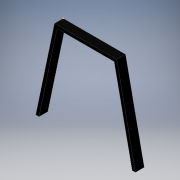
# Autodesk Inventor part: leg
Saved by Autodesk Inventor 2019 (Build 230136000, 136)
## iProperties
Created: 2019-08-11
Part Number: leg
Material: Steel, Galvanized
Document SubType Name: Modeling
Designer: Alex
Density: 7.85 g/cm^3
Appearance: Galvanized
Author: Alex
Autodesk Inventor part; units mm, degrees
ref_plane "YZ Plane" through (0, 0, 0) normal (1, 0, 0) x (0, 1, 0)
ref_plane "XZ Plane" through (0, 0, 0) normal (0, 1, 0) x (-1, 0, 0)
ref_plane "XY Plane" through (0, 0, 0) normal (0, 0, 1) x (1, 0, 0)
sketch "Sketch1" plane through (0, 0, 0) normal (1, 0, 0) x (0, 1, 0)
  point P0 (0, 0)
sketch "Sketch2" plane through (0, 0, 0) normal (0, 0, 1) x (1, 0, 0)
  line L0 (0, 0) -> (500, 0)
  line L1 (650, -710) -> (500, 0)
  line L2 (-150, -710) -> (0, 0)
  line L3 (-22.2287, -226.1612) -> (20.2701, -25)
  line L4 (-22.2287, -226.1612) -> (-124.4482, -710)
  line L5 (572.0133, -461.8084) -> (479.7299, -25)
  line L6 (572.0133, -461.8084) -> (624.4482, -710)
  line L7 (20.2701, -25) -> (479.7299, -25)
  line L8 (-150, -710) -> (-124.4482, -710)
  line L9 (624.4482, -710) -> (650, -710)
  dimension "d0" = 500
  constraints: 20 end point, 5 parallel, 2 horizontal, 1 point on line
  measures "d0" distance of L0.start L0.end
sketch "Sketch3" plane through (0, 0, 0) normal (0, 0, 1) x (1, 0, 0)
  point P0 (0, 0)
extrude "Extrusion1" add sketch "Sketch2" along normal blind 70
body "Solid1"
